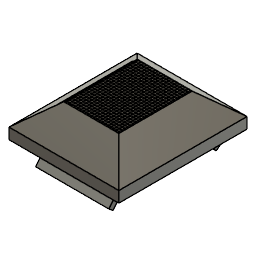
Jetson Orin Nano Case (Autodesk Fusion 360 design; units mm, degrees)
Autodesk Fusion 360 part; units mm, degrees
(part 1 of 4)
sketch "Sketch1" plane through (0, 0, 0) normal (0, 1, 0) x (1, 0, 0)
  line L0 (0, 0) -> (79, 0)
  line L1 (79, 0) -> (79, 100)
  line L2 (79, 100) -> (0, 100)
  line L3 (0, 100) -> (0, 0)
  dimension "d1" = 79
  dimension "d2" = 100
  constraint horizontal L0
  constraint vertical L1
  constraint horizontal L2
  constraint vertical L3
  constraint coincident L0.start L3.end
  measures "d1" distance of L0.start L0.end
  measures "d2" distance of L0.start L2.end
extrude "Extrude1" add sketch "Sketch1" along normal blind 21 makes body 1
sketch "Sketch2" plane through (0, 21, 0) normal (0, 1, 0) x (-1, 0, 0)
  line L0 (0, -100) -> (0, 0)
  line L1 (0, 0) -> (-79, 0)
  line L2 (-79, 0) -> (-79, -100)
  line L3 (-79, -100) -> (0, -100)
  line L4 (-18.6044, -92.1931) -> (-18.6044, -7.1931)
  line L5 (-18.6044, -92.1931) -> (-60.6044, -92.1931)
  line L6 (-60.6044, -92.1931) -> (-60.6044, -7.1931)
  line L7 (-60.6044, -7.1931) -> (-18.6044, -7.1931)
  dimension "d5" = 85
  dimension "d6" = 42
  constraint vertical L4
  constraint perpendicular L4 L5
  constraint perpendicular L5 L6
  constraint perpendicular L4 L7
  measures "d5" distance of L4.start L4.end
  measures "d6" distance of L4.start L5.end
extrude "Extrude2" add sketch "Sketch2" along normal blind 32 separate body contours L4 L5 L6 L7 makes body 2
move_body "Move1" bodies 2 to x (1, 0, 0) y (0, 1, 0) z (0, 0, 1) at (0, 1, 0)
sketch "Sketch3" plane through (0, 21, 0) normal (0, 1, 0) x (-1, 0, 0)
  line L0 (0, -100) -> (0, 0)
  line L1 (0, 0) -> (-79, 0)
  line L2 (-79, 0) -> (-79, -100)
  line L3 (-79, -100) -> (0, -100)
  line L4 (-1, -65.8289) -> (-1, -45.8289)
  line L5 (-1, -85.293) -> (-17.3044, -85.293)
  line L6 (-17.3044, -85.293) -> (-17.3044, -14.9145)
  line L7 (-17.3044, -14.9145) -> (-1, -14.9145)
  line L8 (-1, -14.9145) -> (-1, -85.293)
  constraint horizontal L5
  constraint vertical L6
  constraint horizontal L7
  constraint vertical L8
extrude "Extrude3" add sketch "Sketch3" along normal blind 10 contours L4 L5 L6 L7 L8 bodies 1
sketch "Sketch4" plane through (0, 0, 0) normal (0, 1, 0) x (1, 0, 0)
  line L0 (-20, -20, 1) -> (100, -20, 1)
  line L1 (100, -20, 1) -> (100, 120, 1)
  line L2 (100, 120, 1) -> (-20, 120, 1)
  line L3 (-20, 120, 1) -> (-20, -20, 1)
move_body "Move2" bodies 1 2 to x (1, 0, 0) y (0, 1, 0) z (0, 0, 1) at (0, 3, 0)
extrude "Extrude4" cut sketch "Sketch4" along normal blind 58 contours L0 L1 L2 L3 in plane through (0, 1, 0) normal (0, 1, 0) keep common part bodies 1 2
extrude "Extrude5" add sketch "Sketch4" along normal blind 58 separate body contours L0 L1 L2 L3 in plane through (0, 1, 0) normal (0, 1, 0) makes body 3
extrude "Extrude6" cut sketch "Sketch1" along normal blind 24 bodies 3
extrude "Extrude7" add 1 faces at (93, 1, -33.3333) along direction (0, -1, 0) blind 2 on bodies 3 bodies 3
extrude "Extrude8" cut sketch "Sketch2" along normal blind 35 contours L4 L5 L6 L7 bodies 3
sketch "Sketch5" plane through (-20, 0, 0) normal (-1, 0, 0) x (0, 0, 1)
  line L0 (20, -1) -> (20, 59)
  line L1 (20, 59) -> (-120, 59)
  line L2 (-120, 59) -> (-120, -1)
  line L3 (-120, -1) -> (20, -1)
  line L4 (-90, 59) -> (-120, 35)
  line L5 (-90, -1) -> (-120, 23)
  line L6 (-50, 59) -> (-50, -1)
  line L7 (-10, 59) -> (20, 35)
  line L8 (-10, -1) -> (20, 23)
  constraint coincident L1 L4.start
  constraint coincident L2 L4.end
  constraint coincident L3 L5.start
  constraint coincident L2 L5.end
  constraint midpoint L1 L6.start
  constraint midpoint L3 L6.end
  constraint symmetric L4.start L6 L7.start
  constraint symmetric L4.end L6 L7.end
  constraint symmetric L5.start L6 L8.start
  constraint symmetric L5.end L6 L8.end
sketch "Sketch6" plane through (0, 0, -120) normal (0, 0, -1) x (-1, 0, 0)
  line L0 (20, -1) -> (20, 59)
  line L1 (20, 59) -> (-100, 59)
  line L2 (-100, 59) -> (-100, -1)
  line L3 (-100, -1) -> (20, -1)
  line L4 (20, 35) -> (-10, 59)
  line L5 (20, 23) -> (-10, -1)
  line L6 (-40, 59) -> (-40, -1)
  line L7 (-100, 35) -> (-70, 59)
  line L8 (-100, 23) -> (-70, -1)
  dimension "d25" = 30
  constraint coincident L0 L4.start
  constraint coincident L0 L5.start
  constraint coincident L3 L5.end
  constraint midpoint L1 L6.start
  constraint midpoint L3 L6.end
  constraint symmetric L4.end L6 L7.end
  constraint symmetric L4.start L6 L7.start
  constraint symmetric L5.start L6 L8.start
  constraint symmetric L5.end L6 L8.end
  measures "d25" distance of L0.end L4.end
extrude "Extrude9" cut sketch "Sketch5" against normal blind 130 contours L0 L3 L8 | L0 L1 L7 | L2 L3 L5 | L1 L2 L4 bodies 3
extrude "Extrude10" cut sketch "Sketch6" against normal blind 175 contours L0 L3 L5 | L0 L1 L4 | L2 L3 L8 | L1 L2 L7 bodies 3
sketch "Sketch7" plane through (0, 59, 0) normal (0, 1, 0) x (-1, 0, 0)
  line L0 (-10, -90) -> (-10, -10)
  line L1 (-10, -10) -> (-70, -10)
  line L2 (-70, -10) -> (-70, -90)
  line L3 (-70, -90) -> (-10, -90)
  line L4 (-69, -11) -> (-69.5, -11.866)
  line L5 (-69.5, -11.866) -> (-69, -12.7321)
  line L6 (-69, -12.7321) -> (-68, -12.7321)
  line L7 (-68, -12.7321) -> (-67.5, -11.866)
  line L8 (-67.5, -11.866) -> (-68, -11)
  line L9 (-68, -11) -> (-69, -11)
  line L10 (-65, -11) -> (-66, -11)
  line L11 (-64.5, -11.866) -> (-65, -11)
  line L12 (-65, -12.7321) -> (-64.5, -11.866)
  line L13 (-66, -12.7321) -> (-65, -12.7321)
  line L14 (-66.5, -11.866) -> (-66, -12.7321)
  line L15 (-66, -11) -> (-66.5, -11.866)
  line L16 (-63, -12.7321) -> (-62, -12.7321)
  line L17 (-63.5, -11.866) -> (-63, -12.7321)
  line L18 (-60.5, -11.866) -> (-60, -12.7321)
  line L19 (-60, -12.7321) -> (-59, -12.7321)
  line L20 (-59, -12.7321) -> (-58.5, -11.866)
  line L21 (-60, -11) -> (-60.5, -11.866)
  line L22 (-62, -12.7321) -> (-61.5, -11.866)
  line L23 (-59, -11) -> (-60, -11)
  line L24 (-61.5, -11.866) -> (-62, -11)
  line L25 (-58.5, -11.866) -> (-59, -11)
  line L26 (-63, -11) -> (-63.5, -11.866)
  line L27 (-62, -11) -> (-63, -11)
  line L28 (-57.5, -11.866) -> (-57, -12.7321)
  line L29 (-56, -12.7321) -> (-55.5, -11.866)
  line L30 (-48, -11) -> (-48.5, -11.866)
  line L31 (-47, -12.7321) -> (-46.5, -11.866)
  line L32 (-52.5, -11.866) -> (-53, -11)
  line L33 (-51, -11) -> (-51.5, -11.866)
  line L34 (-54, -12.7321) -> (-53, -12.7321)
  line L35 (-54, -11) -> (-54.5, -11.866)
  line L36 (-57, -11) -> (-57.5, -11.866)
  line L37 (-48, -12.7321) -> (-47, -12.7321)
  line L38 (-55.5, -11.866) -> (-56, -11)
  line L39 (-46.5, -11.866) -> (-47, -11)
  line L40 (-51, -12.7321) -> (-50, -12.7321)
  line L41 (-57, -12.7321) -> (-56, -12.7321)
  line L42 (-54.5, -11.866) -> (-54, -12.7321)
  line L43 (-50, -12.7321) -> (-49.5, -11.866)
  line L44 (-50, -11) -> (-51, -11)
  line L45 (-49.5, -11.866) -> (-50, -11)
  line L46 (-53, -12.7321) -> (-52.5, -11.866)
  line L47 (-53, -11) -> (-54, -11)
  line L48 (-56, -11) -> (-57, -11)
  line L49 (-51.5, -11.866) -> (-51, -12.7321)
  line L50 (-48.5, -11.866) -> (-48, -12.7321)
  line L51 (-47, -11) -> (-48, -11)
  line L52 (-26, -11) -> (-27, -11)
  line L53 (-33, -11) -> (-33.5, -11.866)
  line L54 (-27, -12.7321) -> (-26, -12.7321)
  line L55 (-28.5, -11.866) -> (-29, -11)
  line L56 (-42, -11) -> (-42.5, -11.866)
  line L57 (-25.5, -11.866) -> (-26, -11)
  line L58 (-39, -12.7321) -> (-38, -12.7321)
  line L59 (-35, -12.7321) -> (-34.5, -11.866)
  line L60 (-30, -11) -> (-30.5, -11.866)
  line L61 (-23, -11) -> (-24, -11)
  line L62 (-41, -11) -> (-42, -11)
  line L63 (-33, -12.7321) -> (-32, -12.7321)
  line L64 (-29, -11) -> (-30, -11)
  line L65 (-24, -12.7321) -> (-23, -12.7321)
  line L66 (-42, -12.7321) -> (-41, -12.7321)
  line L67 (-24.5, -11.866) -> (-24, -12.7321)
  line L68 (-23, -12.7321) -> (-22.5, -11.866)
  line L69 (-24, -11) -> (-24.5, -11.866)
  line L70 (-30.5, -11.866) -> (-30, -12.7321)
  line L71 (-29, -12.7321) -> (-28.5, -11.866)
  line L72 (-31.5, -11.866) -> (-32, -11)
  line L73 (-30, -12.7321) -> (-29, -12.7321)
  line L74 (-44, -11) -> (-45, -11)
  line L75 (-35, -11) -> (-36, -11)
  line L76 (-38, -11) -> (-39, -11)
  line L77 (-39.5, -11.866) -> (-39, -12.7321)
  line L78 (-43.5, -11.866) -> (-44, -11)
  line L79 (-39, -11) -> (-39.5, -11.866)
  line L80 (-37.5, -11.866) -> (-38, -11)
  line L81 (-45, -11) -> (-45.5, -11.866)
  line L82 (-36, -11) -> (-36.5, -11.866)
  line L83 (-45, -12.7321) -> (-44, -12.7321)
  line L84 (-36, -12.7321) -> (-35, -12.7321)
  line L85 (-33.5, -11.866) -> (-33, -12.7321)
  line L86 (-44, -12.7321) -> (-43.5, -11.866)
  line L87 (-45.5, -11.866) -> (-45, -12.7321)
  line L88 (-36.5, -11.866) -> (-36, -12.7321)
  line L89 (-34.5, -11.866) -> (-35, -11)
  line L90 (-40.5, -11.866) -> (-41, -11)
  line L91 (-38, -12.7321) -> (-37.5, -11.866)
  line L92 (-41, -12.7321) -> (-40.5, -11.866)
  line L93 (-42.5, -11.866) -> (-42, -12.7321)
  line L94 (-27, -11) -> (-27.5, -11.866)
  line L95 (-32, -12.7321) -> (-31.5, -11.866)
  line L96 (-26, -12.7321) -> (-25.5, -11.866)
  line L97 (-22.5, -11.866) -> (-23, -11)
  line L98 (-27.5, -11.866) -> (-27, -12.7321)
  line L99 (-32, -11) -> (-33, -11)
  line L100 (-17, -11) -> (-18, -11)
  line L101 (-20, -11) -> (-21, -11)
  line L102 (-18.5, -11.866) -> (-18, -12.7321)
  line L103 (-18, -11) -> (-18.5, -11.866)
  line L104 (-21, -11) -> (-21.5, -11.866)
  line L105 (-21.5, -11.866) -> (-21, -12.7321)
  line L106 (-18, -12.7321) -> (-17, -12.7321)
  line L107 (-17, -12.7321) -> (-16.5, -11.866)
  line L108 (-19.5, -11.866) -> (-20, -11)
  line L109 (-20, -12.7321) -> (-19.5, -11.866)
  line L110 (-21, -12.7321) -> (-20, -12.7321)
  line L111 (-16.5, -11.866) -> (-17, -11)
  line L112 (-10.5, -11.866) -> (-11, -11)
  line L113 (-12.5, -11.866) -> (-12, -12.7321)
  line L114 (-11, -12.7321) -> (-10.5, -11.866)
  line L115 (-15, -11) -> (-15.5, -11.866)
  line L116 (-14, -11) -> (-15, -11)
  line L117 (-11, -11) -> (-12, -11)
  line L118 (-14, -12.7321) -> (-13.5, -11.866)
  line L119 (-15, -12.7321) -> (-14, -12.7321)
  line L120 (-12, -11) -> (-12.5, -11.866)
  line L121 (-15.5, -11.866) -> (-15, -12.7321)
  line L122 (-13.5, -11.866) -> (-14, -11)
  line L123 (-12, -12.7321) -> (-11, -12.7321)
  line L124 (-54, -15.7321) -> (-53, -15.7321)
  line L125 (-17, -14) -> (-18, -14)
  line L126 (-12.5, -14.866) -> (-12, -15.7321)
  line L127 (-66.5, -14.866) -> (-66, -15.7321)
  line L128 (-65, -15.7321) -> (-64.5, -14.866)
  line L129 (-15, -14) -> (-15.5, -14.866)
  line L130 (-65, -14) -> (-66, -14)
  line L131 (-23, -15.7321) -> (-22.5, -14.866)
  line L132 (-20, -15.7321) -> (-19.5, -14.866)
  line L133 (-27, -14) -> (-27.5, -14.866)
  line L134 (-11, -15.7321) -> (-10.5, -14.866)
  line L135 (-67.5, -14.866) -> (-68, -14)
  line L136 (-21.5, -14.866) -> (-21, -15.7321)
  line L137 (-53, -15.7321) -> (-52.5, -14.866)
  line L138 (-54, -14) -> (-54.5, -14.866)
  line L139 (-41, -14) -> (-42, -14)
  line L140 (-53, -14) -> (-54, -14)
  line L141 (-48, -14) -> (-48.5, -14.866)
  line L142 (-41, -15.7321) -> (-40.5, -14.866)
  line L143 (-44, -14) -> (-45, -14)
  line L144 (-42, -15.7321) -> (-41, -15.7321)
  line L145 (-43.5, -14.866) -> (-44, -14)
  line L146 (-39.5, -14.866) -> (-39, -15.7321)
  line L147 (-33, -15.7321) -> (-32, -15.7321)
  line L148 (-33.5, -14.866) -> (-33, -15.7321)
  line L149 (-47, -15.7321) -> (-46.5, -14.866)
  line L150 (-32, -15.7321) -> (-31.5, -14.866)
  line L151 (-46.5, -14.866) -> (-47, -14)
  line L152 (-55.5, -14.866) -> (-56, -14)
  line L153 (-32, -14) -> (-33, -14)
  line L154 (-39, -15.7321) -> (-38, -15.7321)
  line L155 (-57.5, -14.866) -> (-57, -15.7321)
  line L156 (-30, -15.7321) -> (-29, -15.7321)
  line L157 (-38, -15.7321) -> (-37.5, -14.866)
  line L158 (-29, -15.7321) -> (-28.5, -14.866)
  line L159 (-36, -15.7321) -> (-35, -15.7321)
  line L160 (-36, -14) -> (-36.5, -14.866)
  line L161 (-31.5, -14.866) -> (-32, -14)
  line L162 (-38, -14) -> (-39, -14)
  line L163 (-30, -14) -> (-30.5, -14.866)
  line L164 (-29, -14) -> (-30, -14)
  line L165 (-34.5, -14.866) -> (-35, -14)
  line L166 (-30.5, -14.866) -> (-30, -15.7321)
  line L167 (-39, -14) -> (-39.5, -14.866)
  line L168 (-35, -14) -> (-36, -14)
  line L169 (-33, -14) -> (-33.5, -14.866)
  line L170 (-37.5, -14.866) -> (-38, -14)
  line L171 (-36.5, -14.866) -> (-36, -15.7321)
  line L172 (-45, -14) -> (-45.5, -14.866)
  line L173 (-56, -14) -> (-57, -14)
  line L174 (-47, -14) -> (-48, -14)
  line L175 (-50, -14) -> (-51, -14)
  line L176 (-51.5, -14.866) -> (-51, -15.7321)
  line L177 (-42, -14) -> (-42.5, -14.866)
  line L178 (-49.5, -14.866) -> (-50, -14)
  line L179 (-57, -14) -> (-57.5, -14.866)
  line L180 (-40.5, -14.866) -> (-41, -14)
  line L181 (-56, -15.7321) -> (-55.5, -14.866)
  line L182 (-48, -15.7321) -> (-47, -15.7321)
  line L183 (-54.5, -14.866) -> (-54, -15.7321)
  line L184 (-44, -15.7321) -> (-43.5, -14.866)
  line L185 (-48.5, -14.866) -> (-48, -15.7321)
  line L186 (-51, -15.7321) -> (-50, -15.7321)
  line L187 (-26, -15.7321) -> (-25.5, -14.866)
  line L188 (-69, -14) -> (-69.5, -14.866)
  line L189 (-68, -14) -> (-69, -14)
  line L190 (-23, -14) -> (-24, -14)
  line L191 (-60, -14) -> (-60.5, -14.866)
  line L192 (-66, -14) -> (-66.5, -14.866)
  line L193 (-21, -15.7321) -> (-20, -15.7321)
  line L194 (-60, -15.7321) -> (-59, -15.7321)
  line L195 (-14, -14) -> (-15, -14)
  line L196 (-60.5, -14.866) -> (-60, -15.7321)
  line L197 (-24, -14) -> (-24.5, -14.866)
  line L198 (-24, -15.7321) -> (-23, -15.7321)
  line L199 (-59, -15.7321) -> (-58.5, -14.866)
  line L200 (-18, -14) -> (-18.5, -14.866)
  line L201 (-62, -14) -> (-63, -14)
  line L202 (-18, -15.7321) -> (-17, -15.7321)
  line L203 (-26, -14) -> (-27, -14)
  line L204 (-17, -15.7321) -> (-16.5, -14.866)
  line L205 (-27.5, -14.866) -> (-27, -15.7321)
  line L206 (-20, -14) -> (-21, -14)
  line L207 (-59, -14) -> (-60, -14)
  line L208 (-69.5, -14.866) -> (-69, -15.7321)
  line L209 (-13.5, -14.866) -> (-14, -14)
  line L210 (-62, -15.7321) -> (-61.5, -14.866)
  line L211 (-15.5, -14.866) -> (-15, -15.7321)
  line L212 (-22.5, -14.866) -> (-23, -14)
  line L213 (-18.5, -14.866) -> (-18, -15.7321)
  line L214 (-12, -15.7321) -> (-11, -15.7321)
  line L215 (-63, -15.7321) -> (-62, -15.7321)
  line L216 (-66, -15.7321) -> (-65, -15.7321)
  line L217 (-12, -14) -> (-12.5, -14.866)
  line L218 (-16.5, -14.866) -> (-17, -14)
  line L219 (-27, -15.7321) -> (-26, -15.7321)
  line L220 (-63, -14) -> (-63.5, -14.866)
  line L221 (-11, -14) -> (-12, -14)
  line L222 (-25.5, -14.866) -> (-26, -14)
  line L223 (-69, -15.7321) -> (-68, -15.7321)
  line L224 (-21, -14) -> (-21.5, -14.866)
  line L225 (-10.5, -14.866) -> (-11, -14)
  line L226 (-19.5, -14.866) -> (-20, -14)
  line L227 (-24.5, -14.866) -> (-24, -15.7321)
  line L228 (-35, -15.7321) -> (-34.5, -14.866)
  line L229 (-58.5, -14.866) -> (-59, -14)
  line L230 (-15, -15.7321) -> (-14, -15.7321)
  line L231 (-28.5, -14.866) -> (-29, -14)
  line L232 (-63.5, -14.866) -> (-63, -15.7321)
  line L233 (-68, -15.7321) -> (-67.5, -14.866)
  line L234 (-14, -15.7321) -> (-13.5, -14.866)
  line L235 (-64.5, -14.866) -> (-65, -14)
  line L236 (-61.5, -14.866) -> (-62, -14)
  line L237 (-57, -15.7321) -> (-56, -15.7321)
  line L238 (-52.5, -14.866) -> (-53, -14)
  line L239 (-50, -15.7321) -> (-49.5, -14.866)
  line L240 (-51, -14) -> (-51.5, -14.866)
  line L241 (-42.5, -14.866) -> (-42, -15.7321)
  line L242 (-45.5, -14.866) -> (-45, -15.7321)
  line L243 (-45, -15.7321) -> (-44, -15.7321)
  line L244 (-45, -20) -> (-45.5, -20.866)
  line L245 (-47, -20) -> (-48, -20)
  line L246 (-43.5, -20.866) -> (-44, -20)
  line L247 (-48, -21.7321) -> (-47, -21.7321)
  line L248 (-60, -17) -> (-60.5, -17.866)
  line L249 (-62, -21.7321) -> (-61.5, -20.866)
  line L250 (-45.5, -20.866) -> (-45, -21.7321)
  line L251 (-63, -20) -> (-63.5, -20.866)
  line L252 (-63.5, -20.866) -> (-63, -21.7321)
  line L253 (-60.5, -20.866) -> (-60, -21.7321)
  line L254 (-47, -21.7321) -> (-46.5, -20.866)
  line L255 (-62, -20) -> (-63, -20)
  line L256 (-47, -18.7321) -> (-46.5, -17.866)
  line L257 (-48.5, -17.866) -> (-48, -18.7321)
  line L258 (-41, -17) -> (-42, -17)
  line L259 (-60.5, -17.866) -> (-60, -18.7321)
  line L260 (-45.5, -17.866) -> (-45, -18.7321)
  line L261 (-58.5, -17.866) -> (-59, -17)
  line L262 (-48, -20) -> (-48.5, -20.866)
  line L263 (-65, -17) -> (-66, -17)
  line L264 (-50, -20) -> (-51, -20)
  line L265 (-65, -18.7321) -> (-64.5, -17.866)
  line L266 (-64.5, -20.866) -> (-65, -20)
  line L267 (-51, -17) -> (-51.5, -17.866)
  line L268 (-56, -18.7321) -> (-55.5, -17.866)
  line L269 (-69, -21.7321) -> (-68, -21.7321)
  line L270 (-68, -21.7321) -> (-67.5, -20.866)
  line L271 (-54, -20) -> (-54.5, -20.866)
  line L272 (-66.5, -20.866) -> (-66, -21.7321)
  line L273 (-50, -18.7321) -> (-49.5, -17.866)
  line L274 (-68, -17) -> (-69, -17)
  line L275 (-65, -21.7321) -> (-64.5, -20.866)
  line L276 (-49.5, -20.866) -> (-50, -20)
  line L277 (-66, -21.7321) -> (-65, -21.7321)
  line L278 (-54, -18.7321) -> (-53, -18.7321)
  line L279 (-67.5, -17.866) -> (-68, -17)
  line L280 (-64.5, -17.866) -> (-65, -17)
  line L281 (-54.5, -17.866) -> (-54, -18.7321)
  line L282 (-67.5, -20.866) -> (-68, -20)
  line L283 (-56, -17) -> (-57, -17)
  line L284 (-53, -18.7321) -> (-52.5, -17.866)
  line L285 (-57, -21.7321) -> (-56, -21.7321)
  line L286 (-66, -18.7321) -> (-65, -18.7321)
  line L287 (-69, -20) -> (-69.5, -20.866)
  line L288 (-66, -20) -> (-66.5, -20.866)
  line L289 (-54, -21.7321) -> (-53, -21.7321)
  line L290 (-56, -20) -> (-57, -20)
  line L291 (-69, -18.7321) -> (-68, -18.7321)
  line L292 (-69.5, -17.866) -> (-69, -18.7321)
  line L293 (-68, -20) -> (-69, -20)
  line L294 (-56, -21.7321) -> (-55.5, -20.866)
  line L295 (-66.5, -17.866) -> (-66, -18.7321)
  line L296 (-66, -17) -> (-66.5, -17.866)
  line L297 (-55.5, -17.866) -> (-56, -17)
  line L298 (-65, -20) -> (-66, -20)
  line L299 (-68, -18.7321) -> (-67.5, -17.866)
  line L300 (-53, -17) -> (-54, -17)
  line L301 (-69, -17) -> (-69.5, -17.866)
  line L302 (-51, -20) -> (-51.5, -20.866)
  line L303 (-69.5, -20.866) -> (-69, -21.7321)
  line L304 (-40.5, -17.866) -> (-41, -17)
  line L305 (-62, -18.7321) -> (-61.5, -17.866)
  line L306 (-42.5, -20.866) -> (-42, -21.7321)
  line L307 (-60, -20) -> (-60.5, -20.866)
  line L308 (-59, -21.7321) -> (-58.5, -20.866)
  line L309 (-42, -20) -> (-42.5, -20.866)
  line L310 (-63, -17) -> (-63.5, -17.866)
  line L311 (-61.5, -20.866) -> (-62, -20)
  line L312 (-41, -21.7321) -> (-40.5, -20.866)
  line L313 (-63, -18.7321) -> (-62, -18.7321)
  line L314 (-63.5, -17.866) -> (-63, -18.7321)
  line L315 (-48.5, -20.866) -> (-48, -21.7321)
  line L316 (-43.5, -17.866) -> (-44, -17)
  line L317 (-12.5, -17.866) -> (-12, -18.7321)
  line L318 (-12, -21.7321) -> (-11, -21.7321)
  line L319 (-12.5, -20.866) -> (-12, -21.7321)
  line L320 (-15.5, -20.866) -> (-15, -21.7321)
  line L321 (-11, -18.7321) -> (-10.5, -17.866)
  line L322 (-18.5, -17.866) -> (-18, -18.7321)
  line L323 (-15.5, -17.866) -> (-15, -18.7321)
  line L324 (-18, -21.7321) -> (-17, -21.7321)
  line L325 (-17, -20) -> (-18, -20)
  line L326 (-11, -17) -> (-12, -17)
  line L327 (-13.5, -17.866) -> (-14, -17)
  line L328 (-14, -18.7321) -> (-13.5, -17.866)
  line L329 (-16.5, -17.866) -> (-17, -17)
  line L330 (-11, -21.7321) -> (-10.5, -20.866)
  line L331 (-10.5, -17.866) -> (-11, -17)
  line L332 (-18, -18.7321) -> (-17, -18.7321)
  line L333 (-21.5, -17.866) -> (-21, -18.7321)
  line L334 (-32, -17) -> (-33, -17)
  line L335 (-31.5, -20.866) -> (-32, -20)
  line L336 (-23, -21.7321) -> (-22.5, -20.866)
  line L337 (-23, -20) -> (-24, -20)
  line L338 (-21, -21.7321) -> (-20, -21.7321)
  line L339 (-30, -17) -> (-30.5, -17.866)
  line L340 (-27, -17) -> (-27.5, -17.866)
  line L341 (-38, -20) -> (-39, -20)
  line L342 (-24.5, -20.866) -> (-24, -21.7321)
  line L343 (-21, -18.7321) -> (-20, -18.7321)
  line L344 (-33.5, -17.866) -> (-33, -18.7321)
  line L345 (-22.5, -17.866) -> (-23, -17)
  line L346 (-29, -17) -> (-30, -17)
  line L347 (-20, -20) -> (-21, -20)
  line L348 (-33, -21.7321) -> (-32, -21.7321)
  line L349 (-27, -21.7321) -> (-26, -21.7321)
  line L350 (-27, -18.7321) -> (-26, -18.7321)
  line L351 (-33.5, -20.866) -> (-33, -21.7321)
  line L352 (-20, -18.7321) -> (-19.5, -17.866)
  line L353 (-26, -17) -> (-27, -17)
  line L354 (-30.5, -20.866) -> (-30, -21.7321)
  line L355 (-30, -18.7321) -> (-29, -18.7321)
  line L356 (-24.5, -17.866) -> (-24, -18.7321)
  line L357 (-32, -20) -> (-33, -20)
  line L358 (-20, -17) -> (-21, -17)
  line L359 (-24, -20) -> (-24.5, -20.866)
  line L360 (-36.5, -20.866) -> (-36, -21.7321)
  line L361 (-23, -18.7321) -> (-22.5, -17.866)
  line L362 (-28.5, -20.866) -> (-29, -20)
  line L363 (-30, -21.7321) -> (-29, -21.7321)
  line L364 (-24, -17) -> (-24.5, -17.866)
  line L365 (-21, -17) -> (-21.5, -17.866)
  line L366 (-27.5, -17.866) -> (-27, -18.7321)
  line L367 (-27.5, -20.866) -> (-27, -21.7321)
  line L368 (-21, -20) -> (-21.5, -20.866)
  line L369 (-32, -18.7321) -> (-31.5, -17.866)
  line L370 (-28.5, -17.866) -> (-29, -17)
  line L371 (-30.5, -17.866) -> (-30, -18.7321)
  line L372 (-25.5, -17.866) -> (-26, -17)
  line L373 (-39, -20) -> (-39.5, -20.866)
  line L374 (-18, -20) -> (-18.5, -20.866)
  line L375 (-15, -21.7321) -> (-14, -21.7321)
  line L376 (-15, -18.7321) -> (-14, -18.7321)
  line L377 (-14, -20) -> (-15, -20)
  line L378 (-29, -18.7321) -> (-28.5, -17.866)
  line L379 (-29, -21.7321) -> (-28.5, -20.866)
  line L380 (-24, -21.7321) -> (-23, -21.7321)
  line L381 (-32, -21.7321) -> (-31.5, -20.866)
  line L382 (-19.5, -20.866) -> (-20, -20)
  line L383 (-31.5, -17.866) -> (-32, -17)
  line L384 (-14, -21.7321) -> (-13.5, -20.866)
  line L385 (-15, -17) -> (-15.5, -17.866)
  line L386 (-16.5, -20.866) -> (-17, -20)
  line L387 (-17, -21.7321) -> (-16.5, -20.866)
  line L388 (-13.5, -20.866) -> (-14, -20)
  line L389 (-17, -18.7321) -> (-16.5, -17.866)
  line L390 (-18.5, -20.866) -> (-18, -21.7321)
  line L391 (-12, -20) -> (-12.5, -20.866)
  line L392 (-11, -20) -> (-12, -20)
  line L393 (-22.5, -20.866) -> (-23, -20)
  line L394 (-33, -17) -> (-33.5, -17.866)
  line L395 (-17, -17) -> (-18, -17)
  line L396 (-14, -17) -> (-15, -17)
  line L397 (-12, -18.7321) -> (-11, -18.7321)
  line L398 (-12, -17) -> (-12.5, -17.866)
  line L399 (-33, -18.7321) -> (-32, -18.7321)
  line L400 (-29, -20) -> (-30, -20)
  line L401 (-20, -21.7321) -> (-19.5, -20.866)
  line L402 (-26, -20) -> (-27, -20)
  line L403 (-25.5, -20.866) -> (-26, -20)
  line L404 (-26, -18.7321) -> (-25.5, -17.866)
  line L405 (-26, -21.7321) -> (-25.5, -20.866)
  line L406 (-10.5, -20.866) -> (-11, -20)
  line L407 (-18, -17) -> (-18.5, -17.866)
  line L408 (-21.5, -20.866) -> (-21, -21.7321)
  line L409 (-30, -20) -> (-30.5, -20.866)
  line L410 (-15, -20) -> (-15.5, -20.866)
  line L411 (-33, -20) -> (-33.5, -20.866)
  line L412 (-45, -18.7321) -> (-44, -18.7321)
  line L413 (-59, -18.7321) -> (-58.5, -17.866)
  line L414 (-63, -21.7321) -> (-62, -21.7321)
  line L415 (-46.5, -20.866) -> (-47, -20)
  line L416 (-58.5, -20.866) -> (-59, -20)
  line L417 (-60, -18.7321) -> (-59, -18.7321)
  line L418 (-42, -21.7321) -> (-41, -21.7321)
  line L419 (-42, -18.7321) -> (-41, -18.7321)
  line L420 (-61.5, -17.866) -> (-62, -17)
  line L421 (-59, -17) -> (-60, -17)
  line L422 (-41, -18.7321) -> (-40.5, -17.866)
  line L423 (-59, -20) -> (-60, -20)
  line L424 (-60, -21.7321) -> (-59, -21.7321)
  line L425 (-40.5, -20.866) -> (-41, -20)
  line L426 (-45, -21.7321) -> (-44, -21.7321)
  line L427 (-62, -17) -> (-63, -17)
  line L428 (-44, -21.7321) -> (-43.5, -20.866)
  line L429 (-48, -18.7321) -> (-47, -18.7321)
  line L430 (-47, -17) -> (-48, -17)
  line L431 (-42, -17) -> (-42.5, -17.866)
  line L432 (-45, -17) -> (-45.5, -17.866)
  line L433 (-44, -18.7321) -> (-43.5, -17.866)
  line L434 (-41, -20) -> (-42, -20)
  line L435 (-46.5, -17.866) -> (-47, -17)
  line L436 (-48, -17) -> (-48.5, -17.866)
  line L437 (-44, -17) -> (-45, -17)
  line L438 (-42.5, -17.866) -> (-42, -18.7321)
  line L439 (-44, -20) -> (-45, -20)
  line L440 (-51, -18.7321) -> (-50, -18.7321)
  line L441 (-54, -17) -> (-54.5, -17.866)
  line L442 (-57.5, -17.866) -> (-57, -18.7321)
  line L443 (-51.5, -17.866) -> (-51, -18.7321)
  line L444 (-55.5, -20.866) -> (-56, -20)
  line L445 (-39.5, -20.866) -> (-39, -21.7321)
  line L446 (-50, -17) -> (-51, -17)
  line L447 (-50, -21.7321) -> (-49.5, -20.866)
  line L448 (-38, -21.7321) -> (-37.5, -20.866)
  line L449 (-37.5, -20.866) -> (-38, -20)
  line L450 (-36, -20) -> (-36.5, -20.866)
  line L451 (-34.5, -20.866) -> (-35, -20)
  line L452 (-36, -17) -> (-36.5, -17.866)
  line L453 (-38, -18.7321) -> (-37.5, -17.866)
  line L454 (-35, -21.7321) -> (-34.5, -20.866)
  line L455 (-39, -18.7321) -> (-38, -18.7321)
  line L456 (-57, -20) -> (-57.5, -20.866)
  line L457 (-39.5, -17.866) -> (-39, -18.7321)
  line L458 (-38, -17) -> (-39, -17)
  line L459 (-36, -18.7321) -> (-35, -18.7321)
  line L460 (-34.5, -17.866) -> (-35, -17)
  line L461 (-36, -21.7321) -> (-35, -21.7321)
  line L462 (-35, -18.7321) -> (-34.5, -17.866)
  line L463 (-35, -17) -> (-36, -17)
  line L464 (-37.5, -17.866) -> (-38, -17)
  line L465 (-24, -18.7321) -> (-23, -18.7321)
  line L466 (-39, -17) -> (-39.5, -17.866)
  line L467 (-57, -17) -> (-57.5, -17.866)
  line L468 (-23, -17) -> (-24, -17)
  line L469 (-35, -20) -> (-36, -20)
  line L470 (-19.5, -17.866) -> (-20, -17)
  line L471 (-36.5, -17.866) -> (-36, -18.7321)
  line L472 (-27, -20) -> (-27.5, -20.866)
  line L473 (-57, -18.7321) -> (-56, -18.7321)
  line L474 (-51.5, -20.866) -> (-51, -21.7321)
  line L475 (-52.5, -17.866) -> (-53, -17)
  line L476 (-51, -21.7321) -> (-50, -21.7321)
  line L477 (-39, -21.7321) -> (-38, -21.7321)
  line L478 (-57.5, -20.866) -> (-57, -21.7321)
  line L479 (-53, -20) -> (-54, -20)
  line L480 (-53, -21.7321) -> (-52.5, -20.866)
  line L481 (-52.5, -20.866) -> (-53, -20)
  line L482 (-54.5, -20.866) -> (-54, -21.7321)
  line L483 (-49.5, -17.866) -> (-50, -17)
  line L484 (-42, -23) -> (-42.5, -23.866)
  line L485 (-48.5, -26.866) -> (-48, -27.7321)
  line L486 (-45, -26) -> (-45.5, -26.866)
  line L487 (-42, -26) -> (-42.5, -26.866)
  line L488 (-48.5, -23.866) -> (-48, -24.7321)
  line L489 (-46.5, -26.866) -> (-47, -26)
  line L490 (-47, -26) -> (-48, -26)
  line L491 (-41, -27.7321) -> (-40.5, -26.866)
  line L492 (-45, -23) -> (-45.5, -23.866)
  line L493 (-45, -27.7321) -> (-44, -27.7321)
  line L494 (-48, -27.7321) -> (-47, -27.7321)
  line L495 (-48, -24.7321) -> (-47, -24.7321)
  line L496 (-48, -26) -> (-48.5, -26.866)
  line L497 (-41, -23) -> (-42, -23)
  line L498 (-40.5, -26.866) -> (-41, -26)
  line L499 (-44, -27.7321) -> (-43.5, -26.866)
  line L500 (-45.5, -26.866) -> (-45, -27.7321)
  line L501 (-44, -24.7321) -> (-43.5, -23.866)
  line L502 (-41, -24.7321) -> (-40.5, -23.866)
  line L503 (-42.5, -23.866) -> (-42, -24.7321)
  line L504 (-41, -26) -> (-42, -26)
  line L505 (-47, -27.7321) -> (-46.5, -26.866)
  line L506 (-47, -24.7321) -> (-46.5, -23.866)
  line L507 (-42, -27.7321) -> (-41, -27.7321)
  line L508 (-43.5, -26.866) -> (-44, -26)
  line L509 (-41, -32) -> (-42, -32)
  line L510 (-48.5, -32.866) -> (-48, -33.7321)
  line L511 (-46.5, -29.866) -> (-47, -29)
  line L512 (-47, -33.7321) -> (-46.5, -32.866)
  line L513 (-47, -29) -> (-48, -29)
  line L514 (-45.5, -32.866) -> (-45, -33.7321)
  line L515 (-44, -33.7321) -> (-43.5, -32.866)
  line L516 (-42, -29) -> (-42.5, -29.866)
  line L517 (-44, -32) -> (-45, -32)
  line L518 (-45, -30.7321) -> (-44, -30.7321)
  line L519 (-65, -30.7321) -> (-64.5, -29.866)
  line L520 (-60, -24.7321) -> (-59, -24.7321)
  line L521 (-35, -32) -> (-36, -32)
  line L522 (-60, -27.7321) -> (-59, -27.7321)
  line L523 (-68, -33.7321) -> (-67.5, -32.866)
  line L524 (-39, -32) -> (-39.5, -32.866)
  line L525 (-38, -30.7321) -> (-37.5, -29.866)
  line L526 (-65, -29) -> (-66, -29)
  line L527 (-39, -29) -> (-39.5, -29.866)
  line L528 (-59, -23) -> (-60, -23)
  line L529 (-34.5, -29.866) -> (-35, -29)
  line L530 (-36.5, -29.866) -> (-36, -30.7321)
  line L531 (-36, -32) -> (-36.5, -32.866)
  line L532 (-38, -27.7321) -> (-37.5, -26.866)
  line L533 (-38, -26) -> (-39, -26)
  line L534 (-39, -33.7321) -> (-38, -33.7321)
  line L535 (-35, -29) -> (-36, -29)
  line L536 (-61.5, -23.866) -> (-62, -23)
  line L537 (-38, -29) -> (-39, -29)
  line L538 (-34.5, -32.866) -> (-35, -32)
  line L539 (-59, -27.7321) -> (-58.5, -26.866)
  line L540 (-66.5, -29.866) -> (-66, -30.7321)
  line L541 (-68, -30.7321) -> (-67.5, -29.866)
  line L542 (-69, -33.7321) -> (-68, -33.7321)
  line L543 (-68, -32) -> (-69, -32)
  line L544 (-66, -32) -> (-66.5, -32.866)
  line L545 (-35, -33.7321) -> (-34.5, -32.866)
  line L546 (-68, -29) -> (-69, -29)
  line L547 (-36, -33.7321) -> (-35, -33.7321)
  line L548 (-67.5, -32.866) -> (-68, -32)
  line L549 (-39, -30.7321) -> (-38, -30.7321)
  line L550 (-36, -30.7321) -> (-35, -30.7321)
  line L551 (-39.5, -29.866) -> (-39, -30.7321)
  line L552 (-59, -26) -> (-60, -26)
  line L553 (-38, -32) -> (-39, -32)
  line L554 (-64.5, -29.866) -> (-65, -29)
  line L555 (-61.5, -26.866) -> (-62, -26)
  line L556 (-35, -30.7321) -> (-34.5, -29.866)
  line L557 (-37.5, -32.866) -> (-38, -32)
  line L558 (-66, -33.7321) -> (-65, -33.7321)
  line L559 (-65, -32) -> (-66, -32)
  line L560 (-35, -26) -> (-36, -26)
  line L561 (-66, -30.7321) -> (-65, -30.7321)
  line L562 (-66.5, -32.866) -> (-66, -33.7321)
  line L563 (-37.5, -29.866) -> (-38, -29)
  line L564 (-63, -26) -> (-63.5, -26.866)
  line L565 (-35, -23) -> (-36, -23)
  line L566 (-60.5, -32.866) -> (-60, -33.7321)
  line L567 (-57.5, -23.866) -> (-57, -24.7321)
  line L568 (-36.5, -32.866) -> (-36, -33.7321)
  line L569 (-38, -33.7321) -> (-37.5, -32.866)
  line L570 (-39.5, -32.866) -> (-39, -33.7321)
  line L571 (-63, -23) -> (-63.5, -23.866)
  line L572 (-36, -29) -> (-36.5, -29.866)
  line L573 (-57, -24.7321) -> (-56, -24.7321)
  line L574 (-58.5, -26.866) -> (-59, -26)
  line L575 (-63.5, -26.866) -> (-63, -27.7321)
  line L576 (-62, -26) -> (-63, -26)
  line L577 (-53, -27.7321) -> (-52.5, -26.866)
  line L578 (-58.5, -23.866) -> (-59, -23)
  line L579 (-60.5, -26.866) -> (-60, -27.7321)
  line L580 (-63.5, -29.866) -> (-63, -30.7321)
  line L581 (-52.5, -23.866) -> (-53, -23)
  line L582 (-51.5, -23.866) -> (-51, -24.7321)
  line L583 (-62, -33.7321) -> (-61.5, -32.866)
  line L584 (-50, -26) -> (-51, -26)
  line L585 (-62, -24.7321) -> (-61.5, -23.866)
  line L586 (-63, -24.7321) -> (-62, -24.7321)
  line L587 (-62, -23) -> (-63, -23)
  line L588 (-51, -27.7321) -> (-50, -27.7321)
  line L589 (-60.5, -23.866) -> (-60, -24.7321)
  line L590 (-60, -23) -> (-60.5, -23.866)
  line L591 (-59, -32) -> (-60, -32)
  line L592 (-59, -33.7321) -> (-58.5, -32.866)
  line L593 (-63.5, -23.866) -> (-63, -24.7321)
  line L594 (-60, -26) -> (-60.5, -26.866)
  line L595 (-53, -26) -> (-54, -26)
  line L596 (-62, -29) -> (-63, -29)
  line L597 (-57.5, -26.866) -> (-57, -27.7321)
  line L598 (-50, -27.7321) -> (-49.5, -26.866)
  line L599 (-54.5, -26.866) -> (-54, -27.7321)
  line L600 (-59, -24.7321) -> (-58.5, -23.866)
  line L601 (-62, -27.7321) -> (-61.5, -26.866)
  line L602 (-63, -27.7321) -> (-62, -27.7321)
  line L603 (-57, -26) -> (-57.5, -26.866)
  line L604 (-53, -24.7321) -> (-52.5, -23.866)
  line L605 (-49.5, -23.866) -> (-50, -23)
  line L606 (-30.5, -26.866) -> (-30, -27.7321)
  line L607 (-30, -23) -> (-30.5, -23.866)
  line L608 (-32, -30.7321) -> (-31.5, -29.866)
  line L609 (-33, -23) -> (-33.5, -23.866)
  line L610 (-24, -33.7321) -> (-23, -33.7321)
  line L611 (-33, -32) -> (-33.5, -32.866)
  line L612 (-23, -32) -> (-24, -32)
  line L613 (-32, -24.7321) -> (-31.5, -23.866)
  line L614 (-21.5, -32.866) -> (-21, -33.7321)
  line L615 (-31.5, -23.866) -> (-32, -23)
  line L616 (-33.5, -32.866) -> (-33, -33.7321)
  line L617 (-28.5, -23.866) -> (-29, -23)
  line L618 (-33.5, -23.866) -> (-33, -24.7321)
  line L619 (-29, -30.7321) -> (-28.5, -29.866)
  line L620 (-24, -30.7321) -> (-23, -30.7321)
  line L621 (-21, -30.7321) -> (-20, -30.7321)
  line L622 (-27, -29) -> (-27.5, -29.866)
  line L623 (-32, -32) -> (-33, -32)
  line L624 (-24, -29) -> (-24.5, -29.866)
  line L625 (-24.5, -29.866) -> (-24, -30.7321)
  line L626 (-30, -30.7321) -> (-29, -30.7321)
  line L627 (-23, -33.7321) -> (-22.5, -32.866)
  line L628 (-26, -33.7321) -> (-25.5, -32.866)
  line L629 (-33, -27.7321) -> (-32, -27.7321)
  line L630 (-20, -30.7321) -> (-19.5, -29.866)
  line L631 (-19.5, -29.866) -> (-20, -29)
  line L632 (-33.5, -26.866) -> (-33, -27.7321)
  line L633 (-20, -32) -> (-21, -32)
  line L634 (-30.5, -23.866) -> (-30, -24.7321)
  line L635 (-30, -27.7321) -> (-29, -27.7321)
  line L636 (-27, -33.7321) -> (-26, -33.7321)
  line L637 (-26, -29) -> (-27, -29)
  line L638 (-32, -26) -> (-33, -26)
  line L639 (-27.5, -29.866) -> (-27, -30.7321)
  line L640 (-31.5, -32.866) -> (-32, -32)
  line L641 (-32, -23) -> (-33, -23)
  line L642 (-21.5, -29.866) -> (-21, -30.7321)
  line L643 (-31.5, -26.866) -> (-32, -26)
  line L644 (-24, -32) -> (-24.5, -32.866)
  line L645 (-33, -26) -> (-33.5, -26.866)
  line L646 (-27.5, -32.866) -> (-27, -33.7321)
  line L647 (-26, -30.7321) -> (-25.5, -29.866)
  line L648 (-29, -23) -> (-30, -23)
  line L649 (-21, -32) -> (-21.5, -32.866)
  line L650 (-22.5, -32.866) -> (-23, -32)
  line L651 (-20, -33.7321) -> (-19.5, -32.866)
  line L652 (-33, -24.7321) -> (-32, -24.7321)
  line L653 (-23, -30.7321) -> (-22.5, -29.866)
  line L654 (-22.5, -29.866) -> (-23, -29)
  line L655 (-26, -32) -> (-27, -32)
  line L656 (-25.5, -32.866) -> (-26, -32)
  line L657 (-24.5, -32.866) -> (-24, -33.7321)
  line L658 (-32, -27.7321) -> (-31.5, -26.866)
  line L659 (-27, -30.7321) -> (-26, -30.7321)
  line L660 (-25.5, -29.866) -> (-26, -29)
  line L661 (-23, -29) -> (-24, -29)
  line L662 (-29, -27.7321) -> (-28.5, -26.866)
  line L663 (-30, -26) -> (-30.5, -26.866)
  line L664 (-27, -32) -> (-27.5, -32.866)
  line L665 (-21, -29) -> (-21.5, -29.866)
  line L666 (-20, -29) -> (-21, -29)
  line L667 (-29, -24.7321) -> (-28.5, -23.866)
  line L668 (-28.5, -26.866) -> (-29, -26)
  line L669 (-21, -33.7321) -> (-20, -33.7321)
  line L670 (-30, -24.7321) -> (-29, -24.7321)
  line L671 (-19.5, -32.866) -> (-20, -32)
  line L672 (-29, -26) -> (-30, -26)
  line L673 (-34.5, -26.866) -> (-35, -26)
  line L674 (-69, -23) -> (-69.5, -23.866)
  line L675 (-65, -33.7321) -> (-64.5, -32.866)
  line L676 (-37.5, -23.866) -> (-38, -23)
  line L677 (-39.5, -26.866) -> (-39, -27.7321)
  line L678 (-69.5, -29.866) -> (-69, -30.7321)
  line L679 (-33.5, -29.866) -> (-33, -30.7321)
  line L680 (-39, -24.7321) -> (-38, -24.7321)
  line L681 (-36, -26) -> (-36.5, -26.866)
  line L682 (-39, -27.7321) -> (-38, -27.7321)
  line L683 (-65, -27.7321) -> (-64.5, -26.866)
  line L684 (-64.5, -32.866) -> (-65, -32)
  line L685 (-35, -24.7321) -> (-34.5, -23.866)
  line L686 (-38, -24.7321) -> (-37.5, -23.866)
  line L687 (-39, -23) -> (-39.5, -23.866)
  line L688 (-69, -29) -> (-69.5, -29.866)
  line L689 (-68, -24.7321) -> (-67.5, -23.866)
  line L690 (-69.5, -32.866) -> (-69, -33.7321)
  line L691 (-35, -27.7321) -> (-34.5, -26.866)
  line L692 (-38, -23) -> (-39, -23)
  line L693 (-36, -24.7321) -> (-35, -24.7321)
  line L694 (-69, -32) -> (-69.5, -32.866)
  line L695 (-36.5, -23.866) -> (-36, -24.7321)
  line L696 (-37.5, -26.866) -> (-38, -26)
  line L697 (-69, -30.7321) -> (-68, -30.7321)
  line L698 (-36, -27.7321) -> (-35, -27.7321)
  line L699 (-39, -26) -> (-39.5, -26.866)
  line L700 (-67.5, -29.866) -> (-68, -29)
  line L701 (-68, -23) -> (-69, -23)
  line L702 (-36.5, -26.866) -> (-36, -27.7321)
  line L703 (-34.5, -23.866) -> (-35, -23)
  line L704 (-66, -29) -> (-66.5, -29.866)
  line L705 (-39.5, -23.866) -> (-39, -24.7321)
  line L706 (-36, -23) -> (-36.5, -23.866)
  line L707 (-66.5, -23.866) -> (-66, -24.7321)
  line L708 (-66.5, -26.866) -> (-66, -27.7321)
  line L709 (-68, -26) -> (-69, -26)
  line L710 (-69.5, -26.866) -> (-69, -27.7321)
  line L711 (-65, -23) -> (-66, -23)
  line L712 (-65, -24.7321) -> (-64.5, -23.866)
  line L713 (-66, -23) -> (-66.5, -23.866)
  line L714 (-30.5, -32.866) -> (-30, -33.7321)
  line L715 (-30, -33.7321) -> (-29, -33.7321)
  line L716 (-30.5, -29.866) -> (-30, -30.7321)
  line L717 (-29, -29) -> (-30, -29)
  line L718 (-69, -26) -> (-69.5, -26.866)
  line L719 (-67.5, -26.866) -> (-68, -26)
  line L720 (-69, -27.7321) -> (-68, -27.7321)
  line L721 (-32, -29) -> (-33, -29)
  line L722 (-66, -24.7321) -> (-65, -24.7321)
  line L723 (-65, -26) -> (-66, -26)
  line L724 (-64.5, -23.866) -> (-65, -23)
  line L725 (-64.5, -26.866) -> (-65, -26)
  line L726 (-28.5, -32.866) -> (-29, -32)
  line L727 (-32, -33.7321) -> (-31.5, -32.866)
  line L728 (-66, -26) -> (-66.5, -26.866)
  line L729 (-68, -27.7321) -> (-67.5, -26.866)
  line L730 (-33, -29) -> (-33.5, -29.866)
  line L731 (-30, -29) -> (-30.5, -29.866)
  line L732 (-29, -33.7321) -> (-28.5, -32.866)
  line L733 (-67.5, -23.866) -> (-68, -23)
  line L734 (-66, -27.7321) -> (-65, -27.7321)
  line L735 (-31.5, -29.866) -> (-32, -29)
  line L736 (-33, -33.7321) -> (-32, -33.7321)
  line L737 (-69.5, -23.866) -> (-69, -24.7321)
  line L738 (-69, -24.7321) -> (-68, -24.7321)
  line L739 (-30, -32) -> (-30.5, -32.866)
  line L740 (-29, -32) -> (-30, -32)
  line L741 (-28.5, -29.866) -> (-29, -29)
  line L742 (-33, -30.7321) -> (-32, -30.7321)
  line L743 (-21, -27.7321) -> (-20, -27.7321)
  line L744 (-25.5, -23.866) -> (-26, -23)
  line L745 (-20, -27.7321) -> (-19.5, -26.866)
  line L746 (-21, -23) -> (-21.5, -23.866)
  line L747 (-23, -24.7321) -> (-22.5, -23.866)
  line L748 (-27, -23) -> (-27.5, -23.866)
  line L749 (-24, -26) -> (-24.5, -26.866)
  line L750 (-24, -23) -> (-24.5, -23.866)
  line L751 (-26, -24.7321) -> (-25.5, -23.866)
  line L752 (-20, -24.7321) -> (-19.5, -23.866)
  line L753 (-26, -23) -> (-27, -23)
  line L754 (-20, -23) -> (-21, -23)
  line L755 (-21.5, -23.866) -> (-21, -24.7321)
  line L756 (-22.5, -26.866) -> (-23, -26)
  line L757 (-24, -27.7321) -> (-23, -27.7321)
  line L758 (-23, -27.7321) -> (-22.5, -26.866)
  line L759 (-23, -23) -> (-24, -23)
  line L760 (-27.5, -23.866) -> (-27, -24.7321)
  line L761 (-27.5, -26.866) -> (-27, -27.7321)
  line L762 (-21, -26) -> (-21.5, -26.866)
  line L763 (-24, -24.7321) -> (-23, -24.7321)
  line L764 (-19.5, -23.866) -> (-20, -23)
  line L765 (-41, -29) -> (-42, -29)
  line L766 (-42, -30.7321) -> (-41, -30.7321)
  line L767 (-47, -32) -> (-48, -32)
  line L768 (-45, -33.7321) -> (-44, -33.7321)
  line L769 (-41, -30.7321) -> (-40.5, -29.866)
  line L770 (-40.5, -29.866) -> (-41, -29)
  line L771 (-45, -29) -> (-45.5, -29.866)
  line L772 (-48.5, -29.866) -> (-48, -30.7321)
  line L773 (-46.5, -32.866) -> (-47, -32)
  line L774 (-45, -32) -> (-45.5, -32.866)
  line L775 (-48, -32) -> (-48.5, -32.866)
  line L776 (-57, -33.7321) -> (-56, -33.7321)
  line L777 (-51, -30.7321) -> (-50, -30.7321)
  line L778 (-54.5, -29.866) -> (-54, -30.7321)
  line L779 (-54, -29) -> (-54.5, -29.866)
  line L780 (-54, -33.7321) -> (-53, -33.7321)
  line L781 (-56, -32) -> (-57, -32)
  line L782 (-51, -32) -> (-51.5, -32.866)
  line L783 (-55.5, -32.866) -> (-56, -32)
  line L784 (-52.5, -32.866) -> (-53, -32)
  line L785 (-49.5, -32.866) -> (-50, -32)
  line L786 (-53, -30.7321) -> (-52.5, -29.866)
  line L787 (-50, -30.7321) -> (-49.5, -29.866)
  line L788 (-50, -32) -> (-51, -32)
  line L789 (-56, -33.7321) -> (-55.5, -32.866)
  line L790 (-62, -30.7321) -> (-61.5, -29.866)
  line L791 (-59, -30.7321) -> (-58.5, -29.866)
  line L792 (-53, -23) -> (-54, -23)
  line L793 (-55.5, -23.866) -> (-56, -23)
  line L794 (-63, -30.7321) -> (-62, -30.7321)
  line L795 (-55.5, -26.866) -> (-56, -26)
  line L796 (-61.5, -32.866) -> (-62, -32)
  line L797 (-60, -30.7321) -> (-59, -30.7321)
  line L798 (-61.5, -29.866) -> (-62, -29)
  line L799 (-56, -27.7321) -> (-55.5, -26.866)
  line L800 (-51, -24.7321) -> (-50, -24.7321)
  line L801 (-58.5, -29.866) -> (-59, -29)
  line L802 (-49.5, -26.866) -> (-50, -26)
  line L803 (-50, -24.7321) -> (-49.5, -23.866)
  line L804 (-54, -24.7321) -> (-53, -24.7321)
  line L805 (-54.5, -23.866) -> (-54, -24.7321)
  line L806 (-56, -26) -> (-57, -26)
  line L807 (-63, -29) -> (-63.5, -29.866)
  line L808 (-60, -33.7321) -> (-59, -33.7321)
  line L809 (-56, -23) -> (-57, -23)
  line L810 (-57, -27.7321) -> (-56, -27.7321)
  line L811 (-60.5, -29.866) -> (-60, -30.7321)
  line L812 (-51, -26) -> (-51.5, -26.866)
  line L813 (-63.5, -32.866) -> (-63, -33.7321)
  line L814 (-51.5, -26.866) -> (-51, -27.7321)
  line L815 (-63, -33.7321) -> (-62, -33.7321)
  line L816 (-60, -32) -> (-60.5, -32.866)
  line L817 (-63, -32) -> (-63.5, -32.866)
  line L818 (-57, -23) -> (-57.5, -23.866)
  line L819 (-54, -27.7321) -> (-53, -27.7321)
  line L820 (-58.5, -32.866) -> (-59, -32)
  line L821 (-50, -23) -> (-51, -23)
  line L822 (-59, -29) -> (-60, -29)
  line L823 (-62, -32) -> (-63, -32)
  line L824 (-60, -29) -> (-60.5, -29.866)
  line L825 (-56, -24.7321) -> (-55.5, -23.866)
  line L826 (-54, -26) -> (-54.5, -26.866)
  line L827 (-52.5, -26.866) -> (-53, -26)
  line L828 (-54, -23) -> (-54.5, -23.866)
  line L829 (-51, -23) -> (-51.5, -23.866)
  line L830 (-44, -30.7321) -> (-43.5, -29.866)
  line L831 (-42, -33.7321) -> (-41, -33.7321)
  line L832 (-48, -30.7321) -> (-47, -30.7321)
  line L833 (-40.5, -32.866) -> (-41, -32)
  line L834 (-44, -29) -> (-45, -29)
  line L835 (-43.5, -32.866) -> (-44, -32)
  line L836 (-42, -32) -> (-42.5, -32.866)
  line L837 (-47, -30.7321) -> (-46.5, -29.866)
  line L838 (-51.5, -29.866) -> (-51, -30.7321)
  line L839 (-54, -32) -> (-54.5, -32.866)
  line L840 (-52.5, -29.866) -> (-53, -29)
  line L841 (-51, -33.7321) -> (-50, -33.7321)
  line L842 (-56, -29) -> (-57, -29)
  line L843 (-55.5, -29.866) -> (-56, -29)
  line L844 (-53, -32) -> (-54, -32)
  line L845 (-57, -32) -> (-57.5, -32.866)
  line L846 (-56, -30.7321) -> (-55.5, -29.866)
  line L847 (-57.5, -29.866) -> (-57, -30.7321)
  line L848 (-54, -30.7321) -> (-53, -30.7321)
  line L849 (-50, -29) -> (-51, -29)
  line L850 (-57, -29) -> (-57.5, -29.866)
  line L851 (-53, -33.7321) -> (-52.5, -32.866)
  line L852 (-50, -33.7321) -> (-49.5, -32.866)
  line L853 (-53, -29) -> (-54, -29)
  line L854 (-51.5, -32.866) -> (-51, -33.7321)
  line L855 (-54.5, -32.866) -> (-54, -33.7321)
  line L856 (-57.5, -32.866) -> (-57, -33.7321)
  line L857 (-49.5, -29.866) -> (-50, -29)
  line L858 (-51, -29) -> (-51.5, -29.866)
  line L859 (-57, -30.7321) -> (-56, -30.7321)
  line L860 (-43.5, -29.866) -> (-44, -29)
  line L861 (-42.5, -32.866) -> (-42, -33.7321)
  line L862 (-45.5, -29.866) -> (-45, -30.7321)
  line L863 (-48, -33.7321) -> (-47, -33.7321)
  line L864 (-41, -33.7321) -> (-40.5, -32.866)
  line L865 (-15.5, -26.866) -> (-15, -27.7321)
  line L866 (-15, -27.7321) -> (-14, -27.7321)
  line L867 (-13.5, -23.866) -> (-14, -23)
  line L868 (-12.5, -26.866) -> (-12, -27.7321)
  line L869 (-14, -24.7321) -> (-13.5, -23.866)
  line L870 (-10.5, -32.866) -> (-11, -32)
  line L871 (-14, -26) -> (-15, -26)
  line L872 (-15, -32) -> (-15.5, -32.866)
  line L873 (-20, -26) -> (-21, -26)
  line L874 (-27, -26) -> (-27.5, -26.866)
  line L875 (-21.5, -26.866) -> (-21, -27.7321)
  line L876 (-26, -27.7321) -> (-25.5, -26.866)
  line L877 (-24.5, -26.866) -> (-24, -27.7321)
  line L878 (-27, -24.7321) -> (-26, -24.7321)
  line L879 (-22.5, -23.866) -> (-23, -23)
  line L880 (-24.5, -23.866) -> (-24, -24.7321)
  line L881 (-27, -27.7321) -> (-26, -27.7321)
  line L882 (-21, -24.7321) -> (-20, -24.7321)
  line L883 (-23, -26) -> (-24, -26)
  line L884 (-26, -26) -> (-27, -26)
  line L885 (-25.5, -26.866) -> (-26, -26)
  line L886 (-15, -33.7321) -> (-14, -33.7321)
  line L887 (-15.5, -29.866) -> (-15, -30.7321)
  line L888 (-11, -27.7321) -> (-10.5, -26.866)
  line L889 (-12, -23) -> (-12.5, -23.866)
  line L890 (-15, -30.7321) -> (-14, -30.7321)
  line L891 (-17, -33.7321) -> (-16.5, -32.866)
  line L892 (-17, -24.7321) -> (-16.5, -23.866)
  line L893 (-18.5, -26.866) -> (-18, -27.7321)
  line L894 (-14, -23) -> (-15, -23)
  line L895 (-18, -27.7321) -> (-17, -27.7321)
  line L896 (-17, -29) -> (-18, -29)
  line L897 (-18, -33.7321) -> (-17, -33.7321)
  line L898 (-15.5, -23.866) -> (-15, -24.7321)
  line L899 (-14, -29) -> (-15, -29)
  line L900 (-15, -29) -> (-15.5, -29.866)
  line L901 (-13.5, -29.866) -> (-14, -29)
  line L902 (-12, -26) -> (-12.5, -26.866)
  line L903 (-14, -33.7321) -> (-13.5, -32.866)
  line L904 (-15, -23) -> (-15.5, -23.866)
  line L905 (-17, -27.7321) -> (-16.5, -26.866)
  line L906 (-12.5, -29.866) -> (-12, -30.7321)
  line L907 (-17, -30.7321) -> (-16.5, -29.866)
  line L908 (-11, -32) -> (-12, -32)
  line L909 (-12.5, -32.866) -> (-12, -33.7321)
  line L910 (-10.5, -26.866) -> (-11, -26)
  line L911 (-18.5, -29.866) -> (-18, -30.7321)
  line L912 (-12, -27.7321) -> (-11, -27.7321)
  line L913 (-11, -33.7321) -> (-10.5, -32.866)
  line L914 (-19.5, -26.866) -> (-20, -26)
  line L915 (-10.5, -23.866) -> (-11, -23)
  line L916 (-14, -30.7321) -> (-13.5, -29.866)
  line L917 (-18, -30.7321) -> (-17, -30.7321)
  line L918 (-13.5, -26.866) -> (-14, -26)
  line L919 (-14, -32) -> (-15, -32)
  line L920 (-16.5, -26.866) -> (-17, -26)
  line L921 (-18, -32) -> (-18.5, -32.866)
  line L922 (-15.5, -32.866) -> (-15, -33.7321)
  line L923 (-11, -26) -> (-12, -26)
  line L924 (-18.5, -23.866) -> (-18, -24.7321)
  line L925 (-14, -27.7321) -> (-13.5, -26.866)
  line L926 (-13.5, -32.866) -> (-14, -32)
  line L927 (-11, -29) -> (-12, -29)
  line L928 (-18, -23) -> (-18.5, -23.866)
  line L929 (-11, -30.7321) -> (-10.5, -29.866)
  line L930 (-12, -24.7321) -> (-11, -24.7321)
  line L931 (-17, -32) -> (-18, -32)
  line L932 (-10.5, -29.866) -> (-11, -29)
  line L933 (-12, -29) -> (-12.5, -29.866)
  line L934 (-12, -33.7321) -> (-11, -33.7321)
  line L935 (-17, -26) -> (-18, -26)
  line L936 (-17, -23) -> (-18, -23)
  line L937 (-18, -29) -> (-18.5, -29.866)
  line L938 (-15, -24.7321) -> (-14, -24.7321)
  line L939 (-18, -26) -> (-18.5, -26.866)
  line L940 (-16.5, -32.866) -> (-17, -32)
  line L941 (-16.5, -29.866) -> (-17, -29)
  line L942 (-12, -32) -> (-12.5, -32.866)
  line L943 (-18, -24.7321) -> (-17, -24.7321)
  line L944 (-11, -24.7321) -> (-10.5, -23.866)
  line L945 (-16.5, -23.866) -> (-17, -23)
  line L946 (-12.5, -23.866) -> (-12, -24.7321)
  line L947 (-11, -23) -> (-12, -23)
  line L948 (-12, -30.7321) -> (-11, -30.7321)
  line L949 (-15, -26) -> (-15.5, -26.866)
  line L950 (-18.5, -32.866) -> (-18, -33.7321)
  line L951 (-45.5, -23.866) -> (-45, -24.7321)
  line L952 (-44, -26) -> (-45, -26)
  line L953 (-40.5, -23.866) -> (-41, -23)
  line L954 (-42.5, -29.866) -> (-42, -30.7321)
  line L955 (-42, -24.7321) -> (-41, -24.7321)
  line L956 (-48, -29) -> (-48.5, -29.866)
  line L957 (-44, -23) -> (-45, -23)
  line L958 (-43.5, -23.866) -> (-44, -23)
  line L959 (-45, -24.7321) -> (-44, -24.7321)
  line L960 (-42.5, -26.866) -> (-42, -27.7321)
  line L961 (-48, -23) -> (-48.5, -23.866)
  line L962 (-47, -23) -> (-48, -23)
  line L963 (-46.5, -23.866) -> (-47, -23)
  line L964 (-44, -50) -> (-45, -50)
  line L965 (-36, -44) -> (-36.5, -44.866)
  line L966 (-48, -53) -> (-48.5, -53.866)
  line L967 (-48, -54.7321) -> (-47, -54.7321)
  line L968 (-45, -54.7321) -> (-44, -54.7321)
  line L969 (-36.5, -47.866) -> (-36, -48.7321)
  line L970 (-44, -56) -> (-45, -56)
  line L971 (-34.5, -41.866) -> (-35, -41)
  line L972 (-47, -53) -> (-48, -53)
  line L973 (-46.5, -50.866) -> (-47, -50)
  line L974 (-39.5, -41.866) -> (-39, -42.7321)
  line L975 (-35, -41) -> (-36, -41)
  line L976 (-38, -47) -> (-39, -47)
  line L977 (-39, -45.7321) -> (-38, -45.7321)
  line L978 (-45, -50) -> (-45.5, -50.866)
  line L979 (-45.5, -56.866) -> (-45, -57.7321)
  line L980 (-36, -41) -> (-36.5, -41.866)
  line L981 (-47, -51.7321) -> (-46.5, -50.866)
  line L982 (-37.5, -41.866) -> (-38, -41)
  line L983 (-47, -50) -> (-48, -50)
  line L984 (-48, -51.7321) -> (-47, -51.7321)
  line L985 (-45, -56) -> (-45.5, -56.866)
  line L986 (-46.5, -56.866) -> (-47, -56)
  line L987 (-39, -44) -> (-39.5, -44.866)
  line L988 (-38, -45.7321) -> (-37.5, -44.866)
  line L989 (-48.5, -50.866) -> (-48, -51.7321)
  line L990 (-48.5, -53.866) -> (-48, -54.7321)
  line L991 (-38, -41) -> (-39, -41)
  line L992 (-48, -50) -> (-48.5, -50.866)
  line L993 (-48, -56) -> (-48.5, -56.866)
  line L994 (-48, -57.7321) -> (-47, -57.7321)
  line L995 (-35, -47) -> (-36, -47)
  line L996 (-47, -56) -> (-48, -56)
  line L997 (-35, -45.7321) -> (-34.5, -44.866)
  line L998 (-45, -53) -> (-45.5, -53.866)
  line L999 (-35, -44) -> (-36, -44)
  line L1000 (-37.5, -47.866) -> (-38, -47)
  line L1001 (-45, -57.7321) -> (-44, -57.7321)
  line L1002 (-35, -48.7321) -> (-34.5, -47.866)
  line L1003 (-48.5, -56.866) -> (-48, -57.7321)
  line L1004 (-46.5, -53.866) -> (-47, -53)
  line L1005 (-36, -45.7321) -> (-35, -45.7321)
  line L1006 (-34.5, -47.866) -> (-35, -47)
  line L1007 (-44, -53) -> (-45, -53)
  line L1008 (-45, -45.7321) -> (-44, -45.7321)
  line L1009 (-48, -45.7321) -> (-47, -45.7321)
  line L1010 (-47, -47) -> (-48, -47)
  line L1011 (-47, -41) -> (-48, -41)
  line L1012 (-45, -44) -> (-45.5, -44.866)
  line L1013 (-48.5, -44.866) -> (-48, -45.7321)
  line L1014 (-37.5, -35.866) -> (-38, -35)
  line L1015 (-39, -35) -> (-39.5, -35.866)
  line L1016 (-44, -44) -> (-45, -44)
  line L1017 (-47, -45.7321) -> (-46.5, -44.866)
  line L1018 (-33, -56) -> (-33.5, -56.866)